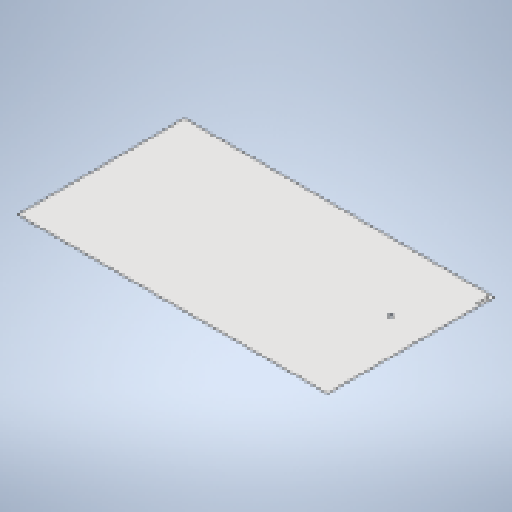
# Autodesk Inventor part: BSH 042 board
Saved by Autodesk Inventor 2025 (Build 290162010, 162A)
## iProperties
Created: 2024-07-23
Part Number: BSH 042 board
Material: 09g2s
Document SubType Name: Sheet Metal
Designer: pokla
Mass: 97143.8 g
Surface Area: 82755 cm^2
Volume: 12375 cm^3
Density: 7.85 g/cm^3
Flat Pattern Width: 274.8 cm
Flat Pattern Length: 147.9 cm
Flat Pattern Area: 40642.9 cm^2
Sheet Metal Rule: AISI304 3mm Die 32
Sheet Metal Width: 2748,000 mm
Sheet Metal Length: 1479,000 mm
Sheet Metal Area: 4064292,000 mm^2
Appearance: Default
Stock Number: БШК 042 борт
Author: admin
Autodesk Inventor part; units mm, degrees
ref_plane "YZ Plane" through (0, 0, 0) normal (1, 0, 0) x (0, 1, 0)
ref_plane "XZ Plane" through (0, 0, 0) normal (0, 1, 0) x (-1, 0, 0)
ref_plane "XY Plane" through (0, 0, 0) normal (0, 0, 1) x (1, 0, 0)
sketch "Sketch1" plane through (0, 0, 0) normal (0, 0, 1) x (1, 0, 0)
  line L0 (-1374, -739.5) -> (1374, -739.5)
  line L1 (1374, -739.5) -> (1374, 739.5)
  line L2 (1374, 739.5) -> (-1374, 739.5)
  line L3 (-1374, 739.5) -> (-1374, -739.5)
  line L4 (-1374, -739.5) -> (1374, 739.5) construction
  line L5 (1374, -739.5) -> (-1374, 739.5) construction
  point P0 (0, 0)
  dimension "d0" = 2748
  dimension "d1" = 1479
  measures "d0" distance of L2.end L1.end
  measures "d1" distance of L1.end L0.end
extrude "Plate1" add sketch "Sketch1" along normal blind 3
sketch "Sketch5" plane through (0, 0, 3) normal (0, 0, 1) x (1, 0, 0)
  line L0 (1349, 714.5) -> (1349, 514.5) construction
  line L1 (1349, 514.5) -> (1334, 514.5) construction
  line L2 (1334, 514.5) -> (1334, 714.5) construction
  line L3 (1334, 714.5) -> (1349, 714.5) construction
  line L4 (1374, 739.5) -> (1374, -739.5) projected
  line L5 (-1374, 739.5) -> (1374, 739.5) projected
  point P0 (0, 0)
  dimension "d26" = 200
  dimension "d27" = 15
  dimension "d28" = 25
  dimension "d29" = 25
  constraints: 2 parallel, 2 other
  measures "d26" distance of L3.end L0.end
  measures "d27" distance between parallel lines of L0 L2
  measures "d28" distance between parallel lines of L4 L0
  measures "d29" distance between parallel lines of L5 L3
mark "Mark1"
sketch "Sketch6" plane through (-1374, -739.5, 3) normal (0, 0, 1) x (1, 0, 0)
  circle A0 centre (2428, 879) radius 20
  line L0 (0, 1479) -> (2748, 1479) projected
  line L1 (2748, 1479) -> (2748, 0) projected
  point P0 (1374, 739.5)
  dimension "d30" = 40
  dimension "d31" = 600
  dimension "d32" = 320
  constraints: 1 centre point
  measures "d30" diameter of A0
  measures "d31" distance from line of L0 A0.centre
  measures "d32" distance from line of L1 A0.centre
extrude "Extrusion2" cut sketch "Sketch6" against normal up to surface (3 mm away)
equation "\"d2\" = Thickness"
equation "\"BendReliefWidth\" = Thickness"
equation "\"BendReliefDepth\" = 0.5 * Thickness"
equation "\"CornerReliefSize\" = 4 * Thickness"
equation "\"MinimumRemnant\" = 2 * Thickness"
equation "\"TransitionRadius\" = BendRadius"
equation "\"JacobiRadiusSize\" = BendRadius"
equation "\"GapSize\" = Thickness"
equation "\"Thickness\" = 3"
equation "\"BendRadius\" = 5"
body "Solid1"
